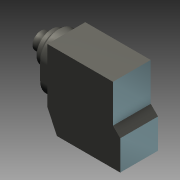
# Autodesk Inventor part: Servo
Saved by Autodesk Inventor 2012 (Build 160160000, 160)
## iProperties
Created: 2013-03-14
Part Number: Servo
Material: Default
Document SubType Name: Modeling
Designer: fixer
Density: 1.86298 g/cm^3
Mass: 17 g
Surface Area: 28.1358 cm^2
Volume: 9.12517 cm^3
Author: fixer
Autodesk Inventor part; units mm, degrees
ref_plane "YZ Plane" through (0, 0, 0) normal (1, 0, 0) x (0, 1, 0)
ref_plane "XZ Plane" through (0, 0, 0) normal (0, 1, 0) x (-1, 0, 0)
ref_plane "XY Plane" through (0, 0, 0) normal (0, 0, 1) x (1, 0, 0)
sketch "Sketch1" plane through (0, 0, 0) normal (0, 0, 1) x (1, 0, 0)
  line L0 (-8.128, -13.081) -> (11.43, -13.081)
  line L1 (11.43, -0.182) -> (11.43, 13.081)
  line L2 (11.43, 13.081) -> (-11.43, 13.081)
  line L3 (-11.43, 13.081) -> (-11.43, -5.969)
  line L4 (11.43, -13.081) -> (-8.128, -13.081)
  line L5 (-8.128, -13.081) -> (-11.43, -5.969)
  line L6 (11.43, -13.081) -> (13.97, -13.081)
  line L7 (13.97, -13.081) -> (13.97, -2.722)
  line L8 (13.97, -2.722) -> (11.43, -0.182)
  point P0 (0, 0)
  point P1 (0, -13.081)
  point P2 (-11.43, 0)
  dimension "d0" = 22.86
  dimension "d1" = 26.162
  dimension "d2" = 19.558
  dimension "d3" = 7.112
  dimension "d4" = 135
  dimension "d5" = 2.54
  constraints: 18 end point, 2 parallel, 2 perpendicular, 1 collinear, 1 horizontal, 1 horizontal alignment, 1 vertical alignment
  measures "d0" distance of L1.end L2.end
  measures "d1" distance of L0.end L1.end
  measures "d2" distance of L0.end L0.start
  measures "d3" distance from line of L0 L3.end
  measures "d4" angle of L8 L7
  measures "d5" distance of L0.end L6.end
extrude "Extrusion1" add sketch "Sketch1" along normal mid plane 13.208
sketch "Sketch2" plane through (-11.43, -5.969, -6.604) normal (-1, 0, 0) x (0, 0, 1)
  line L0 (13.208, 0) -> (13.208, 19.05) projected
  line L1 (0, 19.05) -> (13.208, 19.05) projected
  line L2 (0, 19.05) -> (0, 0) projected
  line L3 (0, 0) -> (13.208, 0) projected
  arc A0 (0, 6.604) -> (13.208, 6.604) centre (6.604, 6.604) ccw
  arc A1 (13.208, 12.446) -> (0, 12.446) centre (6.604, 12.446) ccw
  point P0 (6.604, 5.969)
  constraints: 4 point on circle, 4 tangent, 2 centre point, 2 point on line, 5 other
extrude "Extrusion2" add sketch "Sketch2" along normal blind 3.81 contours A0 L2 A1 L0
chamfer "Chamfer1" distance 1.27 angle 45 4 edges at (-15.24, 13.081, 0) (-15.24, 3.556, 6.604) (-15.24, -5.969, 0) (-15.24, 3.556, -6.604)
sketch "Sketch4" plane through (-15.24, -5.969, -6.604) normal (-1, 0, 0) x (0, 0, 1)
  arc A0 (11.938, 12.446) -> (1.27, 12.446) centre (6.604, 12.446) ccw projected
  circle A1 centre (6.604, 12.446) radius 5.334
  point P0 (6.604, 5.969)
  constraints: 1 centre point, 1 coincident, 1 concentric
extrude "Extrusion3" add sketch "Sketch4" along normal blind 1.27
sketch "Sketch5" plane through (-16.51, 6.477, 0) normal (-1, 0, 0) x (0, 0, 1)
  circle A0 centre (0, 0) radius 5.334 projected
  circle A1 centre (0, 0) radius 2.921
  point P0 (0, -6.477)
  dimension "d15" = 5.842
  constraints: 1 centre point, 1 coincident
  measures "d15" diameter of A1
extrude "Extrusion4" add sketch "Sketch5" along normal blind 3.81 contours A1
body "Solid1"
